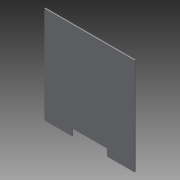
# Autodesk Inventor part: plate
Saved by Autodesk Inventor 2015 (Build 190159000, 159)
## iProperties
Created: 2015-10-02
Part Number: plate
Material: Generic
Document SubType Name: Modeling
Designer: damedin
Density: 1 g/cm^3
Appearance: Default
Author: damedin
Autodesk Inventor part; units mm, degrees
ref_plane "YZ Plane" through (0, 0, 0) normal (1, 0, 0) x (0, 1, 0)
ref_plane "XZ Plane" through (0, 0, 0) normal (0, 1, 0) x (-1, 0, 0)
ref_plane "XY Plane" through (0, 0, 0) normal (0, 0, 1) x (1, 0, 0)
sketch "Sketch1" plane through (0, 0, 0) normal (0, 0, 1) x (1, 0, 0)
  line L0 (-175.444, 104.3404) -> (240.5572, 104.3404)
  line L1 (240.5572, 104.3404) -> (240.5572, -311.6608)
  line L2 (113.5572, -311.6608) -> (-48.444, -311.6608)
  line L3 (-175.444, -311.6608) -> (-175.444, 104.3404)
  line L4 (-48.444, -311.6608) -> (-48.444, -343.6648)
  line L5 (-48.444, -343.6648) -> (-175.444, -343.6648)
  line L6 (-175.444, -343.6648) -> (-175.444, -311.6608)
  line L7 (113.5572, -311.6608) -> (113.5572, -343.6648)
  line L8 (113.5572, -343.6648) -> (240.5572, -343.6648)
  line L9 (240.5572, -343.6648) -> (240.5572, -311.6608)
  point P0 (0, 0)
  dimension "d0" = 416.0012
  dimension "d1" = 416.0012
  dimension "d2" = 127
  dimension "d3" = 127
  dimension "d4" = 162.0012
  dimension "d5" = 32.004
  constraints: 20 end point, 4 parallel, 1 horizontal, 1 perpendicular, 1 point on line
  measures "d0" distance between parallel lines of L2 L0
  measures "d1" distance between parallel lines of L1 L3
  measures "d2" distance between parallel lines of L4 L6
  measures "d3" distance between parallel lines of L9 L7
  measures "d4" distance between parallel lines of L7 L4
  measures "d5" distance between parallel lines of L5 L2
extrude "Extrusion1" add sketch "Sketch1" along normal blind 5.08
body "Solid1"
